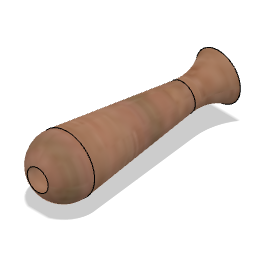
Handle v0 v1 (Autodesk Fusion 360 design; units mm, degrees)
Autodesk Fusion 360 part; units mm, degrees
note: some values were not read from the file. Chosen so that the rebuilt part matches the saved one: a direction.
sketch "Sketch1" plane through (0, 0, 0) normal (1, 0, 0) x (0, 0, -1)
  line L0 (-0.8619, 0) -> (130, 0)
  line L1 (130, 0) -> (130, 15.8604)
  line L2 (104.0572, 9.4893) -> (21.572, 19.8034)
  arc A0 (104.0572, 9.4893) -> (130, 15.8604) centre (108.6974, 46.5989) ccw
  arc A1 (21.572, 19.8034) -> (-0.8619, 0) centre (19.0957, 0) ccw
  constraint horizontal L0
  constraint perpendicular L0 L1
  constraint coincident L0 A1.centre
  constraint tangent L2 A1
  constraint tangent L2 A0
revolve "Revolve1" add sketch "Sketch1" angle 360 about axis through (0, 0, 1.75) along (0, 0, 1) makes body 1
sketch "Sketch2" plane through (0, 0, -130) normal (0, 0, -1) x (-1, 0, 0)
  circle A0 centre (0, 0) radius 15.8604
  circle A1 centre (0, 0) radius 7.5
  circle A2 centre (0, 0) radius 19.8034
  dimension "d2" = 15
  constraint concentric A1 A2
  measures "d2" diameter of A1
extrude "Extrude1" cut sketch "Sketch2" against normal through all contours A1 bodies 1
copy_body "Body->Comp1" bodies 1 removing the originals makes body 2 in component "Component"
component "Component" placed x (1, 0, 0) y (0, 1, 0) z (0, 0, 1) at (0, 0, 0)
